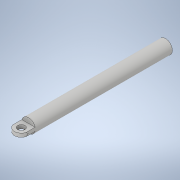
# Autodesk Inventor part: 圓柱3
Saved by Autodesk Inventor 2020 (Build 240168000, 168)
## iProperties
Created: 2021-03-25
Part Number: 圓柱3
Material: 一般
Document SubType Name: Modeling
Designer: cadlab
Density: 1 g/cm^3
Appearance: 預設
Author: cadlab
Autodesk Inventor part; units mm, degrees
ref_plane "YZ Plane" through (0, 0, 0) normal (1, 0, 0) x (0, 1, 0)
ref_plane "XZ Plane" through (0, 0, 0) normal (0, 1, 0) x (-1, 0, 0)
ref_plane "XY Plane" through (0, 0, 0) normal (0, 0, 1) x (1, 0, 0)
sketch "草圖1" plane through (0, 0, 0) normal (0, 0, 1) x (1, 0, 0)
  circle A0 centre (0, 0) radius 9.5
  dimension "d0" = 19
  constraints: 1 centre point, 1 coincident
  measures "d0" diameter of A0
extrude "擠出1" add sketch "草圖1" against normal blind 190
sketch "草圖2" plane through (0, 0, 0) normal (0, 1, 0) x (-1, 0, 0)
  line L0 (-9.5, 0) -> (9.5, 0) projected
  line L1 (9.5, 0) -> (9.5, 10)
  line L2 (-9.5, 0) -> (-9.5, 10)
  arc A0 (9.5, 10) -> (-9.5, 10) centre (0, 10) ccw
  circle A1 centre (0, 10) radius 5
  point P0 (0, 0)
  dimension "d8" = 10
  dimension "d9" = 10
  dimension "d10" = 10
  constraints: 4 end point, 2 centre point, 2 point on circle, 2 vertical, 1 coincident, 1 tangent
  measures "d8" distance of L0.start L2.end
  measures "d9" distance of L0.end L1.end
  measures "d10" diameter of A1
extrude "擠出2" add sketch "草圖2" along normal mid plane 5 contours L2 A0 L1 L0 | A1
delete faces "刪除面1" heal yes whole lump no faces at (9.3386, 2.2259, 0) (9.3386, -2.2259, 0) (-9.3386, 2.2259, 0) (-9.3386, -2.2259, 0)
sketch "草圖3" plane through (0, 2.5, 10) normal (0, 1, 0) x (1, 0, 0)
  circle A0 centre (0, 0) radius 5
  point P0 (0, 10)
  dimension "d11" = 10
  constraints: 1 centre point
  measures "d11" diameter of A0
extrude "擠出3" cut sketch "草圖3" along normal mid plane 10
